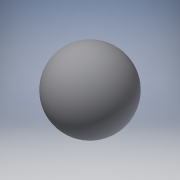
# Autodesk Inventor part: ball
Saved by Autodesk Inventor 2016 (Build 200138000, 138)
## iProperties
Created: 2016-02-03
Part Number: ball
Material: Generic
Document SubType Name: Modeling
Designer: gus
Mass: 8580.25 g
Surface Area: 2026.83 cm^2
Volume: 8580.25 cm^3
Density: 1 g/cm^3
Appearance: Default
Author: gus
Autodesk Inventor part; units mm, degrees
ref_plane "YZ Plane" through (0, 0, 0) normal (1, 0, 0) x (0, 1, 0)
ref_plane "XZ Plane" through (0, 0, 0) normal (0, 1, 0) x (-1, 0, 0)
ref_plane "XY Plane" through (0, 0, 0) normal (0, 0, 1) x (1, 0, 0)
sketch "Sketch1" plane through (0, 0, 0) normal (0, 0, 1) x (1, 0, 0)
  line L0 (0, 0) -> (254, 0)
  line L1 (0, 0) -> (254, 0)
  arc A0 (254, 0) -> (0, 0) centre (127, 0) ccw
  dimension "d0" = 254
  dimension "d2" = 127
  constraints: 4 end point, 2 horizontal, 2 point on circle, 1 centre point, 1 collinear
  measures "d0" distance of L0.start L0.end
  measures "d2" radius of A0
revolve "Revolution1" add sketch "Sketch1" angle 360 about axis through (0, 0, 0) along (1, 0, 0)
body "Solid1"
